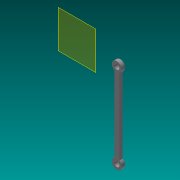
# Autodesk Inventor part: headtilt-long
Saved by Autodesk Inventor 2013 SP2 (Build 170200200, 200)
## iProperties
Created: 2014-11-25
Part Number: headtilt-long
Material: Generic
Document SubType Name: Sheet Metal
Designer: Master
Density: 1 g/cm^3
Sheet Metal Rule: Default
Author: Master
Autodesk Inventor part; units mm, degrees
ref_plane "YZ Plane" through (0, 0, 0) normal (1, 0, 0) x (0, 1, 0)
ref_plane "XZ Plane" through (0, 0, 0) normal (0, 1, 0) x (-1, 0, 0)
ref_plane "XY Plane" through (0, 0, 0) normal (0, 0, 1) x (1, 0, 0)
sketch "Sketch1" plane through (0, 0, 0) normal (0, 0, 1) x (1, 0, 0)
  circle A0 centre (25.1756, 0) radius 1.4986
  circle A1 centre (25.1756, 0) radius 1.4986
  arc A2 (25.1755, -2.8916) -> (25.1758, 2.8915) centre (25.1756, 0) ccw
  arc A3 (26.6742, -2.4729) -> (23.677, -2.4729) centre (25.1756, 0) ccw
  line L0 (23.677, -2.4729) -> (23.677, -46.7314)
  line L1 (23.677, -49.209) -> (26.6742, -49.209)
  line L2 (26.6742, -46.7314) -> (26.6742, -2.4729)
  circle A4 centre (25.1756, -49.209) radius 1.4986
  arc A5 (23.677, -46.7314) -> (26.6742, -46.7314) centre (25.1756, -49.209) ccw
  point P0 (0, 0)
  dimension "d1" = 5.7912
  measures "d1" diameter of A5
ref_plane "Work Plane2" through (0, 0, 0) normal (0, 0, 1) x (1, 0, 0)
extrude "Plate1" add sketch "Sketch1" along normal blind 2
equation "\"BendRadius\" = Thickness"
equation "\"BendReliefWidth\" = Thickness"
equation "\"BendReliefDepth\" = 0.5 * Thickness"
equation "\"CornerReliefSize\" = 4 * Thickness"
equation "\"MinimumRemnant\" = 2 * Thickness"
equation "\"TransitionRadius\" = BendRadius"
equation "\"JacobiRadiusSize\" = BendRadius"
equation "\"GapSize\" = Thickness"
equation "\"d2\" = BendRadius"
equation "\"Thickness\" = 2"
body "Solid1"
